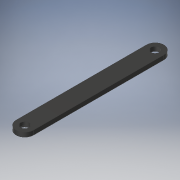
# Autodesk Inventor part: BT001_trajan20_21
Saved by Autodesk Inventor 2022.2 (Build 262287000, 287)
## iProperties
Company: HTBLA Kaindorf
RuleStatus: InUse
Created: 2022-08-07
Part Number: BT001_trajan20_21
Project: Zeichenmaschine_v2
Material: Kunststoff, undurchsichtig Schwarz
Description: gelenk a
Document SubType Name: Modeling
Designer: trajan20
Density: 0.952 g/cm^3
Appearance: Glatt - Schwarz
Mass: 15.0419 g
Surface Area: 84.6918 cm^2
Volume: 15.8003 cm^3
AfterDocNew0: iProperties-Editor_aufrufen
Author: jan
Keywords: 2021
Autodesk Inventor part; units mm, degrees
ref_plane "YZ Plane" through (0, 0, 0) normal (1, 0, 0) x (0, 1, 0)
ref_plane "XZ Plane" through (0, 0, 0) normal (0, 1, 0) x (-1, 0, 0)
ref_plane "XY Plane" through (0, 0, 0) normal (0, 0, 1) x (1, 0, 0)
sketch "Skizze3" plane through (0, 0, 0) normal (0, 0, 1) x (1, 0, 0)
  line L0 (0, 0) -> (-150, 0) construction
  line L1 (0, 10) -> (-150, 10)
  line L2 (-150, -10) -> (0, -10)
  arc A0 (0, -10) -> (0, 10) centre (0, 0) ccw
  arc A1 (-150, 10) -> (-150, -10) centre (-150, 0) ccw
  circle A2 centre (0, 0) radius 5
  circle A3 centre (-150, 0) radius 5
  circle A4 centre (0, 0) radius 4.5
  point P0 (-75, 0)
  dimension "d4" = 150
  dimension "d5" = 20
  dimension "d6" = 10
  dimension "d7" = 10
  dimension "d12" = 9
  constraints: 8 end point, 5 centre point, 4 point on circle, 4 tangent, 3 coincident, 1 horizontal, 1 midpoint, 1 parallel
  measures "d4" distance of L0.end L0.start
  measures "d5" distance between parallel lines of L2 L1
  measures "d6" diameter of A2
  measures "d7" diameter of A3
  measures "d12" diameter of A4
extrude "Extrusion3" add sketch "Skizze3" along normal blind 5 contours A0 L2 A1 L1
extrude "Extrusion4" add sketch "Skizze3" along normal blind 1 contours A2
